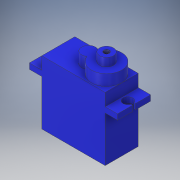
# Autodesk Inventor part: Servo
Saved by Autodesk Inventor 2019.1 (Build 231200000, 200)
## iProperties
Created: 2018-12-04
Part Number: Servo
Material: Generic
Document SubType Name: Modeling
Designer: kfortuna
Density: 1 g/cm^3
Appearance: Default
Author: kfortuna
Autodesk Inventor part; units mm, degrees
ref_plane "YZ Plane" through (0, 0, 0) normal (1, 0, 0) x (0, 1, 0)
ref_plane "XZ Plane" through (0, 0, 0) normal (0, 1, 0) x (-1, 0, 0)
ref_plane "XY Plane" through (0, 0, 0) normal (0, 0, 1) x (1, 0, 0)
sketch "Sketch1" plane through (0, 0, 0) normal (0, 1, 0) x (-1, 0, 0)
  line L0 (12.4948, 19.7938) -> (-10.5052, 19.7938)
  line L1 (-10.5052, 19.7938) -> (-10.5052, 7.7938)
  line L2 (-10.5052, 7.7938) -> (12.4948, 7.7938)
  line L3 (12.4948, 7.7938) -> (12.4948, 19.7938)
  point P0 (0, 0)
  dimension "d0" = 12
  dimension "d1" = 23
  constraints: 8 end point, 2 parallel, 1 horizontal, 1 perpendicular
  measures "d0" distance of L2.end L0.start
  measures "d1" distance of L1.end L2.end
extrude "Extrusion1" add sketch "Sketch1" along normal blind 23
sketch "Sketch2" plane through (10.5052, 0, 19.7938) normal (1, 0, 0) x (0, 0, -1)
  line L0 (0, 0) -> (0, 23) projected
  line L1 (12, 0) -> (12, 23) projected
  line L2 (0, 18.5) -> (12, 18.5)
  line L3 (12, 18.5) -> (12, 16.5)
  line L4 (12, 16.5) -> (0, 16.5)
  line L5 (0, 16.5) -> (0, 18.5)
  line L6 (0, 0) -> (12, 0) projected
  line L7 (0, 23) -> (12, 23) projected
  point P0 (19.7938, 0)
  dimension "d4" = 16.5
  dimension "d7" = 2
  constraints: 8 end point, 2 parallel, 2 point on line, 1 horizontal, 1 perpendicular
  measures "d4" distance between parallel lines of L6 L4
  measures "d7" distance between parallel lines of L2 L4
sketch "Sketch3" plane through (-12.4948, 0, 7.7938) normal (-1, 0, 0) x (0, 0, 1)
  line L0 (0, 16.5) -> (12, 16.5) projected
  line L1 (12, 18.5) -> (0, 18.5) projected
  line L2 (0, 0) -> (0, 23) projected
  line L3 (12, 0) -> (12, 23) projected
  point P0 (-7.7938, 0)
extrude "Extrusion2" add sketch "Sketch3" along normal blind 4.5
extrude "Extrusion3" add sketch "Sketch2" along normal blind 4.5 contours L0 L2 L1 L4
sketch "Sketch4" plane through (10.5052, 18.5, 19.7938) normal (0, 1, 0) x (1, 0, 0)
  arc A0 (3.9271, 6.5) -> (3.9271, 5.5) centre (2.25, 6) ccw
  arc A1 (-26.9271, 5.5) -> (-26.9271, 6.5) centre (-25.25, 6) ccw
  line L0 (0, 12) -> (4.5, 12) projected
  line L1 (-23, 12) -> (-27.5, 12) projected
  line L2 (0, 0) -> (0, 12) projected
  line L3 (4.5, 12) -> (4.5, 0) projected
  line L4 (-23, 12) -> (-23, 0) projected
  line L5 (4.5, 0) -> (4.5, 12) projected
  line L6 (4.5, 6.5) -> (4.5, 6)
  line L7 (-27.5, 12) -> (-27.5, 0) projected
  line L8 (-27.5, 5.5) -> (-26.9271, 5.5)
  line L9 (-26.9271, 6.5) -> (-27.5, 6.5)
  line L10 (-27.5, 6.5) -> (-27.5, 5.5)
  line L11 (0, 0) -> (4.5, 0) projected
  line L12 (4.5, 5.5) -> (3.9271, 5.5)
  line L13 (4.5, 6.5) -> (3.9271, 6.5)
  point P0 (-10.5052, 19.7938)
  dimension "d12" = 3.5
  dimension "d13" = 3.5
  dimension "d15" = 6
  dimension "d16" = 2.25
  dimension "d17" = 2.25
  dimension "d18" = 2.25
  dimension "d22" = 1
  dimension "d26" = 5.5
  dimension "d27" = 5.5
  dimension "d28" = 5.5
  constraints: 12 end point, 4 point on circle, 3 point on line, 2 centre point, 2 horizontal, 1 midpoint, 1 parallel, 1 perpendicular
  measures "d12" diameter of A0
  measures "d13" diameter of A1
  measures "d15" distance from line of L1 A1.centre
  measures "d16" distance from line of L2 A0.centre
  measures "d17" distance from line of L3 A0.centre
  measures "d18" distance from line of L4 A1.centre
  measures "d22" distance between parallel lines of L8 L9
  measures "d26" distance between parallel lines of L11 L12
  measures "d27" distance between parallel lines of L0 L13
  measures "d28" distance between parallel lines of L1 L9
extrude "Extrusion5" cut sketch "Sketch4" against normal blind 4.5 contours L13 L3 L12 A0 | L8 L7 L9 A1
sketch "Sketch6" plane through (0, 23, 0) normal (0, 1, 0) x (1, 0, 0)
  arc A0 (-0.091, -15.8624) -> (-0.091, -11.7252) centre (5.0052, -13.7938) ccw
  arc A1 (-0.091, -11.7252) -> (-0.091, -15.8624) centre (-1.4948, -13.7938) ccw
  line L0 (10.5052, -7.7938) -> (-12.4948, -7.7938) projected
  line L1 (-12.4948, -19.7938) -> (10.5052, -19.7938) projected
  line L2 (10.5052, -19.7938) -> (10.5052, -7.7938) projected
  line L3 (-12.4948, -7.7938) -> (-12.4948, -19.7938) projected
  point P0 (0, 0)
  dimension "d32" = 11
  dimension "d33" = 5
  dimension "d34" = 6
  dimension "d35" = 6
  dimension "d36" = 5.5
  dimension "d37" = 11
  dimension "d38" = 6
  dimension "d39" = 6
  constraints: 4 point on circle, 2 centre point
  measures "d32" diameter of A0
  measures "d33" diameter of A1
  measures "d34" distance from line of L0 A0.centre
  measures "d35" distance from line of L1 A0.centre
  measures "d36" distance from line of L2 A0.centre
  measures "d37" distance from line of L3 A1.centre
  measures "d38" distance from line of L0 A1.centre
  measures "d39" distance from line of L1 A1.centre
extrude "Extrusion6" add sketch "Sketch6" along normal blind 4 contours A1 A0
sketch "Sketch7" plane through (0, 27, 0) normal (0, 1, 0) x (1, 0, 0)
  circle A0 centre (5.0052, -13.7938) radius 2.5
  line L0 (10.5052, -7.7938) -> (-12.4948, -7.7938) projected
  line L1 (-12.4948, -19.7938) -> (10.5052, -19.7938) projected
  line L2 (10.5052, -13.7938) -> (10.5052, -7.7938) projected
  point P0 (0, 0)
  dimension "d42" = 5
  dimension "d43" = 6
  dimension "d44" = 6
  dimension "d45" = 5.5
  constraints: 1 centre point
  measures "d42" diameter of A0
  measures "d43" distance from line of L0 A0.centre
  measures "d44" distance from line of L1 A0.centre
  measures "d45" distance from line of L2 A0.centre
extrude "Extrusion7" add sketch "Sketch7" along normal blind 3
sketch "Sketch8" plane through (5.0052, 30, 13.7938) normal (0, 1, 0) x (1, 0, 0)
  circle A0 centre (0, 0) radius 1
  point P0 (-5.0052, 13.7938)
  dimension "d48" = 2
  constraints: 1 centre point
  measures "d48" diameter of A0
extrude "Extrusion8" cut sketch "Sketch8" against normal blind 3
thread "Thread1" size "M2x0.4" class "6H" standard "ANSI Metric M Profile" full length
body "Solid1"
